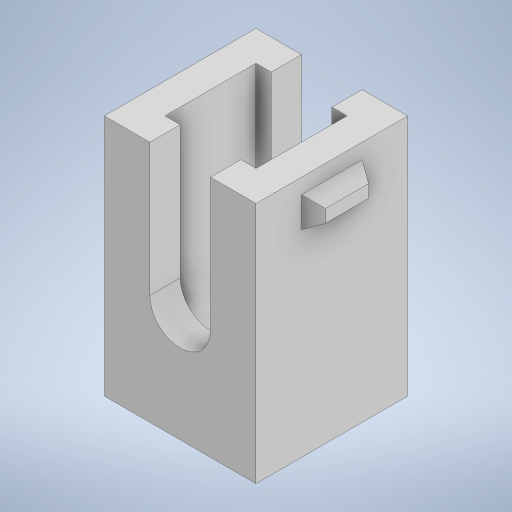
# Autodesk Inventor part: snapfit_part_v03
Saved by Autodesk Inventor 2023 (Build 270158000, 158)
## iProperties
Created: 2022-03-20
Part Number: snapfit_part_v03
Material: Generic
Document SubType Name: Modeling
Designer: LIMlab
Density: 1 g/cm^3
Appearance: Default
Author: LIMlab
Autodesk Inventor part; units mm, degrees
ref_plane "YZ Plane" through (0, 0, 0) normal (1, 0, 0) x (0, 1, 0)
ref_plane "XZ Plane" through (0, 0, 0) normal (0, 1, 0) x (-1, 0, 0)
ref_plane "XY Plane" through (0, 0, 0) normal (0, 0, 1) x (1, 0, 0)
sketch "Sketch1" plane through (0, 0, 0) normal (0, 1, 0) x (-1, 0, 0)
  line L0 (-2.5, 2.5) -> (2.5, 2.5)
  line L1 (2.5, 2.5) -> (2.5, -2.5)
  line L2 (2.5, -2.5) -> (-2.5, -2.5)
  line L3 (-2.5, -2.5) -> (-2.5, 2.5)
  line L4 (-2.5, 2.5) -> (2.5, -2.5) construction
  line L5 (2.5, 2.5) -> (-2.5, -2.5) construction
  point P0 (0, 0)
  dimension "d0" = 5
  dimension "d1" = 5
  constraints: 12 end point, 2 midpoint, 2 parallel, 1 horizontal, 1 perpendicular
  measures "d0" distance of L0.end L1.end
  measures "d1" distance of L1.end L2.end
extrude "Extrusion1" add sketch "Sketch1" along normal blind 8
shell "Shell1" thickness 1 removed faces 1 at (-0.8333, 8, -0.8333)
sketch "Sketch9" plane through (2.5, 0, 2.5) normal (1, 0, 0) x (0, 0, -1)
  line L0 (1.5, 6.5) -> (3.5, 6.5)
  line L1 (3.5, 6.5) -> (3.5, 7.5)
  line L2 (3.5, 7.5) -> (1.5, 7.5)
  line L3 (1.5, 7.5) -> (1.5, 6.5)
  line L4 (1.5, 6.5) -> (3.5, 7.5) construction
  line L5 (3.5, 6.5) -> (1.5, 7.5) construction
  line L6 (0, 8) -> (5, 8) projected
  point P0 (2.5, 0)
  point P1 (2.5, 7)
  dimension "d10" = 1
  dimension "d14" = 2
  dimension "d15" = 1
  constraints: 12 end point, 2 midpoint, 2 parallel, 1 horizontal, 1 perpendicular
  measures "d10" distance from line of point (2.5, 7) L6
  measures "d14" distance of L1.end L2.end
  measures "d15" distance of L0.end L1.end
extrude "Extrusion4" add sketch "Sketch9" along normal blind 0.5 draft -30
sketch "Sketch10" plane through (-2.5, 0, -2.5) normal (-1, 0, 0) x (0, 0, 1)
  line L0 (1.5, 6.5) -> (3.5, 6.5)
  line L1 (3.5, 6.5) -> (3.5, 7.5)
  line L2 (3.5, 7.5) -> (1.5, 7.5)
  line L3 (1.5, 7.5) -> (1.5, 6.5)
  line L4 (1.5, 6.5) -> (3.5, 7.5) construction
  line L5 (3.5, 6.5) -> (1.5, 7.5) construction
  line L6 (0, 8) -> (5, 8) projected
  point P0 (2.5, 0)
  point P1 (2.5, 7)
  dimension "d13" = 1
  dimension "d16" = 2
  dimension "d17" = 1
  constraints: 12 end point, 2 midpoint, 2 parallel, 1 horizontal, 1 perpendicular
  measures "d13" distance from line of point (2.5, 7) L6
  measures "d16" distance of L1.end L2.end
  measures "d17" distance of L0.end L1.end
extrude "Extrusion5" add sketch "Sketch10" along normal blind 0.5 draft -30
sketch "Sketch11" plane through (2.5, 0, -2.5) normal (0, 0, -1) x (-1, 0, 0)
  line L0 (2.5, 7.862) -> (2.5, 3.6245) construction
  line L1 (1.5, 7.862) -> (1.5, 3.6245)
  line L2 (3.5, 3.6245) -> (3.5, 7.862)
  arc A0 (3.5, 7.862) -> (1.5, 7.862) centre (2.5, 7.862) ccw
  arc A1 (1.5, 3.6245) -> (3.5, 3.6245) centre (2.5, 3.6245) ccw
  point P0 (2.5, 0)
  point P1 (2.5, 5.7432)
  dimension "d20" = 2
  constraints: 8 end point, 4 point on circle, 4 tangent, 2 centre point, 1 midpoint, 1 parallel, 1 vertical
  measures "d20" diameter of A1
extrude "Extrusion6" cut sketch "Sketch11" against normal through all
sketch "Sketch12" plane through (2.5, 0, -2.5) normal (0, 0, -1) x (-1, 0, 0)
  line L0 (1.5, 7.862) -> (1.5, 3.6245) projected
  line L1 (1.5, 7.862) -> (3.5, 7.862)
  line L2 (3.5, 7.862) -> (3.5, 10.4679)
  line L3 (3.5, 10.4679) -> (1.5, 10.4679)
  line L4 (1.5, 10.4679) -> (1.5, 7.862)
  point P0 (2.5, 0)
  dimension "d23" = 2
  constraints: 8 end point, 2 parallel, 1 horizontal, 1 perpendicular
  measures "d23" distance of L3.end L2.end
extrude "Extrusion7" cut sketch "Sketch12" against normal through all
equation "\"d16\" = d14"
equation "\"d17\" = d15"
body "Solid1"
